07b46ed1-3801-45ad-9f42-5adfffb4e1c7 (Autodesk Fusion 360 design; units mm, degrees)
Autodesk Fusion 360 part; units mm, degrees
sketch "Sketch3" plane through (0, 0, 0) normal (0, 0, 1) x (1, 0, 0)
  circle A0 centre (0, 0) radius 1.5
  circle A1 centre (0, 0) radius 0.7
  dimension "d7" = 3
  measures "d7" diameter of A0
extrude "Extrude2" add sketch "Sketch3" against normal blind 1.4 contours A0 | A1 picked at (1.227749, -0.074521) picked at (0.479259, -0.127273) makes body 1
sketch "Sketch4" plane through (0, 0, -1.4) normal (0, 0, -1) x (1, 0, 0)
  circle A0 centre (0, 0) radius 1.5
  line L0 (0.057374, 0.748359) -> (-0.619411, 0.423867)
  line L1 (-0.619411, 0.423867) -> (-0.676785, -0.324492)
  line L2 (-0.676785, -0.324492) -> (-0.057374, -0.748359)
  line L3 (-0.057374, -0.748359) -> (0.619411, -0.423867)
  line L4 (0.619411, -0.423867) -> (0.676785, 0.324492)
  line L5 (0.676785, 0.324492) -> (0.057374, 0.748359)
  dimension "d10" = 0.65
  dimension "d11" = 1.3
  measures "d10" distance of A0.centre L5
  measures "d11" distance of L1 L4
extrude "Extrude3" cut sketch "Sketch4" against normal blind 0.975 contours L0 L1 L2 L3 L4 L5 picked at (0, 0) bodies 1
sketch "Sketch5" plane through (0, 0, -1.4) normal (0, 0, -1) x (1, 0, 0)
  line L0 (-0.619411, 0.423867) -> (0.057374, 0.748359)
  line L1 (0.057374, 0.748359) -> (0.676785, 0.324492)
  line L2 (0.676785, 0.324492) -> (0.619411, -0.423867)
  line L3 (0.619411, -0.423867) -> (-0.057374, -0.748359)
  line L4 (-0.057374, -0.748359) -> (-0.676785, -0.324492)
  line L5 (-0.676785, -0.324492) -> (-0.619411, 0.423867)
  circle A0 centre (0, 0) radius 1.5
  circle A1 centre (0, 0) radius 0.750555
extrude "Extrude4" cut sketch "Sketch5" against normal blind 0.5 draft -45 contours L0 A1 | L0 L1 L2 L3 L4 L5 | L5 A1 | L1 A1 | L4 A1 | L2 A1 | L3 A1 picked at (-0.370452, 0.561226) picked at (0.019125, 0.249453) picked at (-0.671262, -0.040208) picked at (0.42841, 0.527471) picked at (-0.451674, -0.498196) picked at (0.653968, -0.148676) picked at (0.205614, -0.640259) bodies 1
chamfer "Chamfer1" distance 0.09 angle 45 2 edges at (-1.398491, 0.542423, -1.4) (-1.398491, -0.542423, 0) on bodies 1
sketch "Sketch14" plane through (0, 0, 0) normal (0, 0, 1) x (1, 0, 0)
  circle A0 centre (0, 0) radius 0.7
sketch "Sketch15" plane through (0, 0, 0) normal (0, 0, 1) x (1, 0, 0)
  circle A0 centre (0, 0) radius 0.7
sketch "Sketch16" plane through (0, 0, 0) normal (0, 0, 1) x (1, 0, 0)
  circle A0 centre (0, 0) radius 0.7
extrude "Extrude5" add sketch "Sketch16" along normal blind 10 separate body contours A0 picked at (-0.222967, 0.38619) makes body 2
thread "Thread10" "ISO Metric profile 1.7 M1.7x0.35 4g6g" major diameter 1.6385 minor diameter 1.2501 pitch 0.35 angle 60 modelled left hand crest width 0.04375 on face at (0.69913, -0.034892, 6.666667) crest through (0.81925, 0, -0.021875) on bodies 2
equation "d7 = HeadDia"
equation "d8 = -HeadHt"
equation "d10 = ( DriveSize / 2 )"
equation "d12 = -( DriveSize ) * 0.75"
equation "d16 = HeadDia * 0.03"
equation "ShaftDia = 1.4 mm"
equation "ShaftLength = 3 mm"
equation "HeadDia = 3 mm"
equation "HeadHt = 1.4 mm"
equation "DriveSize = 1.3 mm"
equation "Pitch = 0.3 mm"
